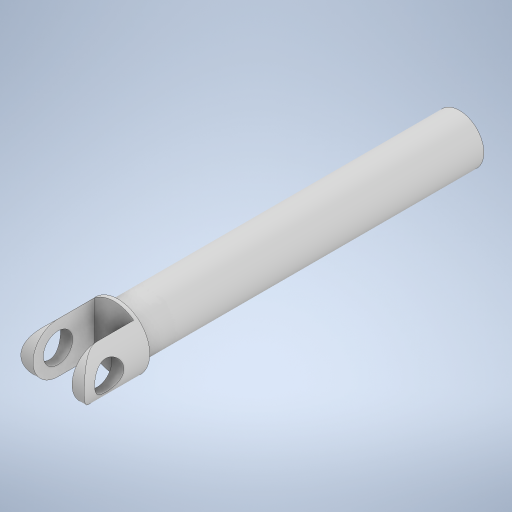
# Autodesk Inventor part: czlon_1
Saved by Autodesk Inventor 2023 (Build 270158000, 158)
## iProperties
Created: 2023-04-01
Part Number: czlon_1
Material: Ogólny
Document SubType Name: Modeling
Designer: krzys
Density: 1 g/cm^3
Appearance: Domyślna
Author: krzys
Autodesk Inventor part; units mm, degrees
ref_plane "YZ Plane" through (0, 0, 0) normal (1, 0, 0) x (0, 1, 0)
ref_plane "XZ Plane" through (0, 0, 0) normal (0, 1, 0) x (-1, 0, 0)
ref_plane "XY Plane" through (0, 0, 0) normal (0, 0, 1) x (1, 0, 0)
sketch "Szkic1" plane through (0, 0, 0) normal (0, 0, 1) x (1, 0, 0)
  circle A0 centre (0, 0) radius 50
  circle A1 centre (0, 0) radius 46
  circle A2 centre (0, 0) radius 31.5
  circle A3 centre (-28.991378, 28.991378) radius 4
  circle A4 centre (-28.991378, -28.991378) radius 4
  circle A5 centre (28.991378, 28.991378) radius 4
  circle A6 centre (28.991378, -28.991378) radius 4
  dimension "d0" = 100
  dimension "d1" = 92
  dimension "d2" = 63
  dimension "d4" = 8
  dimension "d5" = 8
  dimension "d6" = 8
  dimension "d7" = 8
  constraints: 7 centre point, 3 coincident
  measures "d0" diameter of A0
  measures "d1" diameter of A1
  measures "d2" diameter of A2
  measures "d4" diameter of A3
  measures "d5" diameter of A4
  measures "d6" diameter of A5
  measures "d7" diameter of A6
extrude "Wyciągnięcie proste1" add sketch "Szkic1" along normal blind 4 contours A1
extrude "Wyciągnięcie proste2" add sketch "Szkic1" along normal blind 700 contours A0
sketch "Szkic2" plane through (0, 0, 700) normal (0, 0, 1) x (1, 0, 0)
  circle A0 centre (0, 0) radius 65
  line L0 (40, -51.234754) -> (40, 51.234754)
  line L1 (-40, 51.234754) -> (-40, -51.234754)
  line L2 (-40, -65) -> (40, 65) construction
  line L3 (40, -65) -> (-40, 65) construction
  line L4 (50, 41.533119) -> (50, -41.533119)
  line L5 (-50, -41.533119) -> (-50, 41.533119)
  line L6 (-50, 41.533119) -> (50, -41.533119) construction
  line L7 (50, 41.533119) -> (-50, -41.533119) construction
  dimension "d12" = 130
  constraints: 16 end point, 5 point on circle, 4 midpoint, 2 parallel, 1 centre point, 1 coincident
  measures "d12" diameter of A0
extrude "Wyciągnięcie proste3" add sketch "Szkic2" along normal blind 8
extrude "Wyciągnięcie proste4" add sketch "Szkic2" along normal blind 150 contours A0 L4 | L4 A0 L0 | L1 A0 L5 | L5 A0
sketch "Szkic3" plane through (-40, -51.234754, 708) normal (1, 0, 0) x (0, 0, -1)
  circle A0 centre (-75, 51.234754) radius 30
  arc A1 (-75, 102.469508) -> (-75, 0) centre (-75, 51.234754) ccw
  line L0 (0, 102.469508) -> (-142, 102.469508)
  line L1 (0, 102.469508) -> (0, 0)
  line L2 (-71, 102.469508) -> (0, 102.469508)
  line L3 (0, 0) -> (0, -13.765246)
  line L4 (0, 102.469508) -> (0, 0)
  line L5 (0, 0) -> (-75, 0)
  line L6 (0, 0) -> (-142, 0)
  line L7 (-142, 102.469508) -> (-142, 0)
  line L8 (-75, 102.469508) -> (-142, 102.469508)
  line L9 (-142, 102.469508) -> (-142, 0)
  line L10 (-142, 0) -> (-75, 0)
  point P0 (708, 51.234754)
  dimension "d19" = 60
  constraints: 12 end point, 3 collinear, 2 centre point, 2 point on circle, 2 point on line, 1 coincident, 1 horizontal, 1 midpoint, 1 perpendicular, 1 tangent
  measures "d19" diameter of A0
extrude "Wyciągnięcie proste5" cut sketch "Szkic3" along normal blind 150 and the other way blind 75 contours A1 L6 L7 L0
extrude "Wyciągnięcie proste6" cut sketch "Szkic3" along normal blind 150 and the other way blind 75 contours A0
